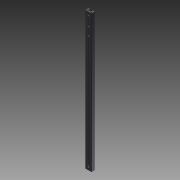
# Autodesk Inventor part: HFSFIN5-1020-432-Z5-XA10-XB40-XC65-XD422
Saved by Autodesk Inventor 2011 SP1 (Build 150282100, 282)
## iProperties
Created: 2016-04-06
Part Number: HFSFIN5-1020-432-Z5-XA10-XB40-XC65-XD422
Catalog Web Link: www.cadenas.de
Description: HFSFIN-Flat Aluminum Extrusions - HFSFIN
Vendor: MISUMI
Document SubType Name: Modeling
Designer: psAdmin
Manufacturer: MISUMI
Mass: 55.7304 g
Surface Area: 434.655 cm^2
Volume: 55.7304 cm^3
Density: 1 g/cm^3
Category: PARTsolutions
Company: MISUMI
Title: HFSFIN5-1020-432-Z5-XA10-XB40-XC65-XD422
Author: Cadenas PARTsolutions
Comments: Flat Aluminum Extrusions - HFSFIN
PSOL_IDENT_0: {$CADENAS_DATA\23d-libs\misumi\metric\38_al_extrusions_blackets\hfsfin.prj},283 {VTYP=3D},{NB=HFSFIN
PSOL_IDENT_1: 5-1020-432-Z5-XA10-XB40-XC65-XD422},{LINA=HFSFIN5-1020-432-Z5-XA10-XB40-XC65-XD422},{NN=HFSFIN},{DAT
PSOL_IDENT_2: E=13.01.2016 07:28:10},{GEOMDATE=25.12.2015 01:20:09},{VERSION=},{LINEID=10},{LINESUBID=-1},{WBVAR=L
PSOL_IDENT_3: ,ALT1,Z,ZN,ZXA,ZXB,ZXC,ZXD,ZXE,ALT2,D,DN,DXA,DXB,DXC,DXD,DXE}  {NB=HFSFIN5-1020-432-Z5-XA10-XB40-XC6
PSOL_IDENT_4: 5-XD422},{LINA=HFSFIN5-1020-432-Z5-XA10-XB40-XC65-XD422},{KT=DUMMY},{PN=HFSFIN5-1020-432-Z5-XA10-XB4
PSOL_IDENT_5: 0-XC65-XD422},{TPS=HFSFIN5-1020},{L=432},{ALT1=Z},{ALT1ALG='','w/o Z (Counterboring)','Z','with Z (C
PSOL_IDENT_6: ounterboring)'},{ALT1PN=-Z5-XA10-XB40-XC65-XD422},{Z=5},{ZALG=3,4,5,6,8},{DD=5.5},{DD1=9.5},{ZN=4},{
PSOL_IDENT_7: ZNALG=[1,2,3,4,5]},{ZNMAX=37},{ZXA=10.0},{ZXB=40.0},{ZXC=65.0},{ZXD=422.0},{ZXE=0.0},{ZXAMIN=7},{ZXB
PSOL_IDENT_8: MIN=21.5},{ZXCMIN=51.5},{ZXDMIN=76.5},{ZXEMIN=433.5},{ZXAMAX=390.5},{ZXBMAX=402},{ZXCMAX=413.5},{ZXD
PSOL_IDENT_9: MAX=425},{ZXEMAX=425},{ZXAALG=[7:390.5/0.5]},{ZXBALG=[21.5:402/0.5]},{ZXCALG=[51.5:413.5/0.5]},{ZXDA
PSOL_IDENT_10: LG=[76.5:425/0.5]},{ZXEALG=[0]},{ALT2=},{ALT2ALG='','N/A'},{ALT2PN=},{D=0.0},{DALG=0},{DN=0},{DNALG=
PSOL_IDENT_11: [0]},{DNMAX=37},{DXA=0.0},{DXB=0.0},{DXC=0.0},{DXD=0.0},{DXE=0.0},{DXAMIN=7},{DXBMIN=11.5},{DXCMIN=1
PSOL_IDENT_12: 1.5},{DXDMIN=11.5},{DXEMIN=11.5},{DXAMAX=436.5},{DXBMAX=448},{DXCMAX=459.5},{DXDMAX=471},{DXEMAX=425
PSOL_IDENT_13: },{DXAALG=[0]},{DXBALG=[0]},{DXCALG=[0]},{DXDALG=[0]},{DXEALG=[0]},{CL=7},{HDIS=11.5},{DEG=30}
NN: HFSFIN
NT: Flat Aluminum Extrusions - HFSFIN
NB: HFSFIN5-1020-432-Z5-XA10-XB40-XC65-XD422
NBSYN: $PN.
LINA: HFSFIN5-1020-432-Z5-XA10-XB40-XC65-XD422
PN: HFSFIN5-1020-432-Z5-XA10-XB40-XC65-XD422
TPS: HFSFIN5-1020
L: 432
ALT1: with Z (Counterboring)
Z: 5
DD: 5.5
DD1: 9.5
ZN: 4
ZXA: 10.0
ZXB: 40.0
ZXC: 65.0
ZXD: 422.0
ZXE: 0.0
ALT2: N/A
D: 0.0
DN: 0
DXA: 0.0
DXB: 0.0
DXC: 0.0
DXD: 0.0
DXE: 0.0
SUPPLIER: MISUMI
ARTICLENO: HFSFIN5-1020-432-Z5-XA10-XB40-XC65-XD422
BOMINFO: HFSFIN5-1020-432-Z5-XA10-XB40-XC65-XD422
CREATOR: CADENAS GmbH
Autodesk Inventor part; units mm, degrees
ref_plane "YZ Plane" through (0, 0, 0) normal (1, 0, 0) x (0, 1, 0)
ref_plane "XZ Plane" through (0, 0, 0) normal (0, 1, 0) x (-1, 0, 0)
ref_plane "XY Plane" through (0, 0, 0) normal (0, 0, 1) x (1, 0, 0)
sketch "_____1" plane through (0, 0, 0) normal (0, 0, 1) x (1, 0, 0)
  arc A0 (-10, 1) -> (-9, 0) centre (-9, 1) ccw
  line L0 (-9, 0) -> (-0.5196, 0)
  line L1 (-0.5196, 0) -> (0, 0.3)
  line L2 (0, 0.3) -> (0.5196, 0)
  line L3 (0.5196, 0) -> (9, 0)
  arc A1 (9, 0) -> (10, 1) centre (9, 1) ccw
  line L4 (10, 1) -> (10, 9)
  arc A2 (10, 9) -> (9, 10) centre (9, 9) ccw
  line L5 (9, 10) -> (-9, 10)
  arc A3 (-9, 10) -> (-10, 9) centre (-9, 9) ccw
  line L6 (-10, 9) -> (-10, 1)
  constraints: 14 end point, 8 point on circle, 4 centre point
extrude "Extrusion1" add sketch "_____1" against normal blind 432
sketch "_____2" plane through (0, 0, 0) normal (0, 0, 1) x (1, 0, 0)
  line L0 (-6, 8) -> (-6, 7)
  line L1 (-6, 7) -> (-4.15, 5)
  line L2 (-4.15, 5) -> (-4.15, 4.4)
  arc A0 (-4.15, 4.4) -> (-3.75, 4) centre (-3.75, 4.4) ccw
  line L3 (-3.75, 4) -> (-0.5196, 4)
  line L4 (-0.5196, 4) -> (0, 3.7)
  line L5 (0, 3.7) -> (0.5196, 4)
  line L6 (0.5196, 4) -> (3.75, 4)
  arc A1 (3.75, 4) -> (4.15, 4.4) centre (3.75, 4.4) ccw
  line L7 (4.15, 4.4) -> (4.15, 5)
  line L8 (4.15, 5) -> (6, 7)
  line L9 (6, 7) -> (6, 8)
  line L10 (6, 8) -> (3, 8)
  line L11 (3, 8) -> (3, 10)
  line L12 (3, 10) -> (-3, 10)
  line L13 (-3, 10) -> (-3, 8)
  line L14 (-3, 8) -> (-6, 8)
  constraints: 30 end point, 4 point on circle, 2 centre point
extrude "Extrusion2" cut sketch "_____2" against normal blind 432
sketch "Sketch3" plane through (0, 0, -432) normal (0, 0, -1) x (-1, 0, 0)
  point P0 (-7, 2.6)
hole "Hole1" at (7, 2.6, -432) direction (0, 0, 1) diameter 3.2 depth 432
sketch "Sketch4" plane through (0, 0, -432) normal (0, 0, -1) x (-1, 0, 0)
  point P0 (7, 2.6)
hole "Hole2" at (-7, 2.6, -432) direction (0, 0, 1) diameter 3.2 depth 432
sketch "_____5" plane through (0, 0, 0) normal (1, 0, 0) x (0, 0, -1)
  line L0 (10, 0) -> (10, 10)
  line L1 (10, 10) -> (14.75, 10)
  line L2 (14.75, 10) -> (14.75, 4)
  line L3 (14.75, 4) -> (12.75, 4)
  line L4 (12.75, 4) -> (12.75, 0)
  line L5 (12.75, 0) -> (10, 0)
  line L6 (10, 0) -> (10, 10)
  constraints: 14 end point
revolve "Revolution1" cut sketch "_____5" angle 360 about axis through (0, 0, -10) along (0, -1, 0)
sketch "_____6" plane through (0, 0, 0) normal (1, 0, 0) x (0, 0, -1)
  line L0 (40, 0) -> (40, 10)
  line L1 (40, 10) -> (44.75, 10)
  line L2 (44.75, 10) -> (44.75, 7)
  line L3 (44.75, 7) -> (42.75, 7)
  line L4 (42.75, 7) -> (42.75, 0)
  line L5 (42.75, 0) -> (40, 0)
  line L6 (40, 0) -> (40, 10)
  constraints: 14 end point
revolve "Revolution2" cut sketch "_____6" angle 360 about axis through (0, 0, -40) along (0, -1, 0)
sketch "_____7" plane through (0, 0, 0) normal (1, 0, 0) x (0, 0, -1)
  line L0 (65, 0) -> (65, 10)
  line L1 (65, 10) -> (69.75, 10)
  line L2 (69.75, 10) -> (69.75, 7)
  line L3 (69.75, 7) -> (67.75, 7)
  line L4 (67.75, 7) -> (67.75, 0)
  line L5 (67.75, 0) -> (65, 0)
  line L6 (65, 0) -> (65, 10)
  constraints: 14 end point
revolve "Revolution3" cut sketch "_____7" angle 360 about axis through (0, 0, -65) along (0, -1, 0)
sketch "_____8" plane through (0, 0, 0) normal (1, 0, 0) x (0, 0, -1)
  line L0 (422, 0) -> (422, 10)
  line L1 (422, 10) -> (426.75, 10)
  line L2 (426.75, 10) -> (426.75, 7)
  line L3 (426.75, 7) -> (424.75, 7)
  line L4 (424.75, 7) -> (424.75, 0)
  line L5 (424.75, 0) -> (422, 0)
  line L6 (422, 0) -> (422, 10)
  constraints: 14 end point
revolve "Revolution4" cut sketch "_____8" angle 360 about axis through (0, 0, -422) along (0, -1, 0)
body "Solid1"
